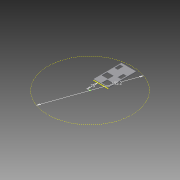
# Autodesk Inventor part: Molecule Chopper
Saved by Autodesk Inventor 2015 (Build 190159000, 159)
## iProperties
Created: 2014-07-07
Part Number: Molecule Chopper
Material: Generic
Document SubType Name: Modeling
Designer: I Rabey
Density: 1 g/cm^3
Appearance: Default
Author: I Rabey
Autodesk Inventor part; units mm, degrees
ref_plane "YZ Plane" through (0, 0, 0) normal (1, 0, 0) x (0, 1, 0)
ref_plane "XZ Plane" through (0, 0, 0) normal (0, 1, 0) x (-1, 0, 0)
ref_plane "XY Plane" through (0, 0, 0) normal (0, 0, 1) x (1, 0, 0)
sketch "Sketch2" plane through (0, 0, 0) normal (0, 1, 0) x (-1, 0, 0)
  line L0 (-17, 32.5) -> (17, 32.5)
  line L1 (17, 32.5) -> (17, -32.5)
  line L2 (17, -32.5) -> (-17, -32.5)
  line L3 (-17, -32.5) -> (-17, 32.5)
  line L4 (-17, 32.5) -> (17, -32.5) construction
  line L5 (17, 32.5) -> (-17, -32.5) construction
  line L6 (0, 30.5) -> (-15, 30.5)
  line L7 (-15, 30.5) -> (-15, 17.5)
  line L8 (-15, 17.5) -> (0, 17.5)
  line L9 (0, 17.5) -> (0, 30.5)
  line L10 (0, 15.5) -> (15, 15.5)
  line L11 (15, 15.5) -> (15, 2.5)
  line L12 (15, 2.5) -> (0, 2.5)
  line L13 (0, 2.5) -> (0, 15.5)
  line L14 (-7.5, 0.5) -> (-15, 0.5)
  line L15 (-15, 0.5) -> (-15, -12.5)
  line L16 (-15, -12.5) -> (-7.5, -12.5)
  line L17 (-7.5, -12.5) -> (-7.5, 0.5)
  line L18 (15, -14.5) -> (7.5, -14.5)
  line L19 (7.5, -14.5) -> (7.5, -27.5)
  line L20 (7.5, -27.5) -> (15, -27.5)
  line L21 (15, -27.5) -> (15, -14.5)
  point P0 (0, 0)
  dimension "d35" = 34
  dimension "d36" = 65
  dimension "d37" = 15
  dimension "d38" = 13
  dimension "d39" = 15
  dimension "d40" = 13
  dimension "d41" = 2
  dimension "d42" = 2
  dimension "d43" = 0
  dimension "d44" = 2
  dimension "d45" = 7.5
  dimension "d46" = 13
  dimension "d47" = 7.5
  dimension "d48" = 2
  dimension "d49" = 7.5
  dimension "d50" = 13
  dimension "d51" = 2
  dimension "d52" = 2
  constraints: 44 end point, 10 parallel, 5 horizontal, 5 perpendicular, 2 midpoint, 1 point on line
  measures "d35" distance of L1.end L2.end
  measures "d36" distance of L0.end L1.end
  measures "d37" distance of L8.end L7.end
  measures "d38" distance of L7.end L6.end
  measures "d39" distance of L11.end L12.end
  measures "d40" distance of L10.end L11.end
  measures "d41" distance between parallel lines of L0 L6
  measures "d42" distance between parallel lines of L10 L8
  measures "d43" distance from line of point (0, 0) L9
  measures "d44" distance between parallel lines of L3 L7
  measures "d45" distance of L16.end L15.end
  measures "d46" distance of L15.end L14.end
  measures "d47" distance from line of point (0, 0) L17
  measures "d48" distance between parallel lines of L14 L12
  measures "d49" distance of L20.end L19.end
  measures "d50" distance of L19.end L18.end
  measures "d51" distance between parallel lines of L18 L16
  measures "d52" distance between parallel lines of L1 L21
extrude "Extrusion4" add sketch "Sketch2" along normal blind 2
sketch "Sketch3" plane through (0, 0, 0) normal (0, 1, 0) x (-1, 0, 0)
  circle A0 centre (0, 57.5) radius 97.6 construction
  line L0 (17, 32.5) -> (-17, 32.5) projected
  point P0 (0, 0)
  dimension "d55" = 195.2
  dimension "d56" = 25
  constraints: 1 centre point
  measures "d55" diameter of A0
  measures "d56" distance from line of L0 A0.centre
body "Solid4"
